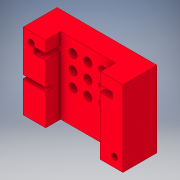
# Autodesk Inventor part: EDMO1-0_Cover
Saved by Autodesk Inventor 2019 (Build 230136000, 136)
## iProperties
Created: 2016-10-24
Part Number: EDMO1-0_Cover
Material: PLA
Document SubType Name: Modeling
Designer: Lucas
Density: 1.29985 g/cm^3
Appearance: Plastic Vinyl
Mass: 17.4066 g
Surface Area: 60.0154 cm^2
Volume: 13.3912 cm^3
Author: Lucas
Autodesk Inventor part; units mm, degrees
ref_plane "YZ Plane" through (0, 0, 0) normal (1, 0, 0) x (0, 1, 0)
ref_plane "XZ Plane" through (0, 0, 0) normal (0, 1, 0) x (-1, 0, 0)
ref_plane "XY Plane" through (0, 0, 0) normal (0, 0, 1) x (1, 0, 0)
sketch "Sketch2" plane through (0, 0, 0) normal (0, 0, 1) x (1, 0, 0)
  line L0 (0, 0) -> (42, 0)
  line L1 (42, 0) -> (42, 32)
  line L2 (42, 32) -> (0, 32)
  line L3 (0, 32) -> (0, 0)
  dimension "d0" = 42
  dimension "d1" = 32
  constraints: 8 end point, 2 parallel, 1 horizontal, 1 perpendicular
  measures "d0" distance of L2.end L1.end
  measures "d1" distance of L1.end L0.end
extrude "Cover_Body" add sketch "Sketch2" along normal blind 15.8
sketch "Sketch4" plane through (0, 0, 15.8) normal (0, 0, 1) x (1, 0, 0)
  line L0 (42, 32) -> (0, 32) projected
  line L1 (0, 32) -> (0, 0) projected
  line L2 (4.5, 24.6) -> (9.5, 24.6)
  line L3 (32.5, 24.6) -> (37.5, 24.6)
  line L4 (42, 0) -> (42, 32) projected
  line L5 (0, 0) -> (42, 0) projected
  line L6 (4.5, 24.6) -> (4.5, 27.1)
  line L7 (4.5, 27.1) -> (9.5, 27.1)
  line L8 (9.5, 27.1) -> (9.5, 32)
  line L9 (37.5, 27.1) -> (37.5, 24.6)
  line L10 (37.5, 27.1) -> (32.5, 27.1)
  line L11 (32.5, 27.1) -> (32.5, 32)
  line L12 (9.5, 32) -> (32.5, 32)
  line L13 (21, 36.5125) -> (21, -47.625) construction
  line L14 (32.5, 24.6) -> (32.5, 0)
  line L15 (9.5, 24.6) -> (9.5, 0)
  line L16 (9.5, 0) -> (32.5, 0)
  point P0 (4.9935, 32)
  point P1 (37, 32)
  dimension "d6" = 5
  dimension "d14" = 2.5
  dimension "d15" = 2.5
  dimension "d22" = 42
  dimension "d23" = 21
  dimension "d24" = 23
  dimension "d28" = 5
  dimension "d118" = 23
  dimension "d119" = 11.5
  dimension "d120" = 11.5
  dimension "d121" = 24.6
  constraints: 26 end point, 6 point on line, 5 perpendicular, 4 collinear, 3 horizontal, 2 vertical
  measures "d6" distance of L2.start L2.end
  measures "d14" distance of L2.start L6.end
  measures "d15" distance of L9.start L3.end
  measures "d22" distance between parallel lines of L4 L1
  measures "d23" distance between parallel lines of L13 L1
  measures "d24" distance between parallel lines of L11 L8
  measures "d28" distance of L9.start L10.end
  measures "d118" distance between parallel lines of L15 L14
  measures "d119" distance between parallel lines of L13 L11
  measures "d120" distance between parallel lines of L13 L14
  measures "d121" distance of L3.start L14.end
extrude "Servo_Opening" cut sketch "Sketch4" against normal blind 6.3 contours L11 L10 L9 L3 L14 L5 L15 L2 L6 L7 L8 L0
sketch "Sketch5" plane through (0, 0, 15.8) normal (0, 0, 1) x (1, 0, 0)
  line L0 (0, 32) -> (0, 0) projected
  line L1 (0, 13.2) -> (0, 14.7)
  line L2 (-29.647, 13.95) -> (54.8226, 13.95) construction
  line L3 (0, 0) -> (42, 0) projected
  line L4 (0, 14.7) -> (9.5, 14.7)
  line L5 (9.5, 14.7) -> (9.5, 13.2)
  line L6 (9.5, 13.2) -> (0, 13.2)
  line L7 (9.5, 0) -> (9.5, 24.6) projected
  line L8 (9.5, 32) -> (0, 32) projected
  dimension "d97" = 1.5
  dimension "d131" = 13.2
  constraints: 10 end point, 2 horizontal, 1 collinear, 1 perpendicular, 1 point on line, 1 other
  measures "d97" distance of L4.end L5.end
  measures "d131" distance between parallel lines of L6 L3
extrude "Cable_Opening" cut sketch "Sketch5" against normal blind 2.5 contours L4 L5 L6 L0
sketch "Sketch6" plane through (0, 0, 15.8) normal (0, 0, 1) x (1, 0, 0)
  circle A0 centre (3.5, 28) radius 1.25
  circle A1 centre (38.5, 28) radius 1.25 construction
  circle A2 centre (38.5, 4) radius 1.25
  circle A3 centre (3.5, 4) radius 1.25 construction
  line L0 (21, 34.35) -> (21, -13.275) construction
  line L1 (-20.6375, 16) -> (66.675, 16) construction
  line L2 (42, 0) -> (42, 32) projected
  line L3 (0, 32) -> (0, 0) projected
  line L4 (9.5, 32) -> (0, 32) projected
  line L5 (0, 0) -> (42, 0) projected
  point P0 (42, 12.35)
  point P1 (0, 12.35)
  dimension "d29" = 2.5
  dimension "d30" = 2.5
  dimension "d31" = 2.5
  dimension "d32" = 2.5
  dimension "d33" = 42
  dimension "d34" = 21
  dimension "d35" = 32
  dimension "d36" = 16
  dimension "d37" = 35
  dimension "d38" = 17.5
  dimension "d39" = 24
  dimension "d40" = 12
  constraints: 4 centre point, 4 end point, 2 horizontal alignment, 2 vertical alignment, 1 horizontal
  measures "d29" diameter of A0
  measures "d30" diameter of A1
  measures "d31" diameter of A2
  measures "d32" diameter of A3
  measures "d33" distance between parallel lines of L2 L3
  measures "d34" distance between parallel lines of L0 L3
  measures "d35" distance between parallel lines of L4 L5
  measures "d36" distance between parallel lines of L4 L1
  measures "d37" distance of A1.centre A0.centre
  measures "d38" distance from line of L0 A0.centre
  measures "d39" distance of A3.centre A0.centre
  measures "d40" distance from line of L1 A2.centre
extrude "Holes_Mounting_Screws" cut sketch "Sketch6" against normal up to surface (15.8 mm away)
sketch "Sketch16" plane through (0, 0, 0) normal (0, 0, -1) x (-1, 0, 0)
  circle A0 centre (-38.5, 4) radius 2.25
  circle A1 centre (-3.5, 28) radius 2.25
  circle A2 centre (-38.5, 4) radius 1.25 projected
  circle A3 centre (-3.5, 28) radius 1.25 projected
  dimension "d99" = 4.5
  dimension "d100" = 4.5
  constraints: 2 centre point, 2 concentric
  measures "d99" diameter of A0
  measures "d100" diameter of A1
extrude "Pocket_Mounting_Screws" cut sketch "Sketch16" against normal blind 9
sketch "Sketch17" plane through (0, 0, 9.5) normal (0, 0, 1) x (1, 0, 0)
  circle A0 centre (14.75, 26.6) radius 1.75
  line L0 (9.5, 32) -> (32.5, 32) projected
  line L1 (9.5, 27.1) -> (9.5, 32) projected
  point P0 (0, 0)
  dimension "d105" = 3.5
  dimension "d106" = 5.4
  dimension "d107" = 5.25
  constraints: 1 centre point
  measures "d105" diameter of A0
  measures "d106" distance from line of L0 A0.centre
  measures "d107" distance from line of L1 A0.centre
extrude "Heat_Dissipation_Hole" cut sketch "Sketch17" against normal up to surface (9.5 mm away)
pattern_linear "Pattern_Heat_Dissipation_Hole" count 3 spacing 6.25 along (1, 0, 0) count 3 spacing 6.25 along (0, -1, 0) of "Heat_Dissipation_Hole"
sketch "Sketch25" plane through (0, 0, 0) normal (0, 0, -1) x (-1, 0, 0)
  line L0 (0, 32) -> (0, 0) projected
  line L1 (-42, 32) -> (-32.5, 32) projected
  line L2 (0, 0) -> (-42, 0)
  line L3 (-42, 0) -> (-42, 32)
  line L4 (-42, 32) -> (0, 32)
  line L5 (0, 32) -> (0, 0)
  constraints: 8 end point, 2 parallel, 1 horizontal, 1 perpendicular
extrude "Material_Reduction_Optional" cut sketch "Sketch25" against normal blind 1.5
equation "\"d15\" = d14"
equation "\"d23\" = 0.5 * d22"
equation "\"d28\" = d6"
equation "\"d120\" = 0.5 * d118"
equation "\"d34\" = 0.5 * d33"
equation "\"d36\" = 0.5 * d35"
equation "\"d38\" = 0.5 * d37"
equation "\"d40\" = 0.5 * d39"
equation "\"d99\" = d101"
equation "\"d100\" = d101"
equation "\"d101\" = 4.5"
body "Solid1"
